Autodesk Inventor part; units mm, degrees
(part 2 of 2)
  spline S298 degree 2 poles (63.8368, 1.8656) (63.9127, 1.8656) (64.0147, 1.785) (64.0692, 1.6) (64.0977, 1.5668) knots 0 0 0 1 2 3 3 3
  spline S299 degree 2 poles (64.0977, 1.5668) (64.1593, 1.5004) (64.4676, 1.3676) (64.6503, 1.3676) knots 0 0 0 1 2 2 2
  spline S300 degree 2 poles (64.6503, 1.3676) (64.9372, 1.3676) (65.1222, 1.5004) knots 0 0 0 1 1 1
  spline S301 degree 2 poles (65.1222, 1.5004) (65.2384, 1.5834) (65.2384, 1.702) knots 0 0 0 1 1 1
  spline S302 degree 2 poles (65.2384, 1.702) (65.2384, 1.7826) (65.127, 1.9226) (64.9989, 1.9676) knots 0 0 0 1 2 2 2
  spline S303 degree 2 poles (64.9989, 1.9676) (64.9159, 1.9985) (64.6265, 2.053) knots 0 0 0 1 1 1
  spline S304 degree 2 poles (64.6265, 2.053) (64.2755, 2.1194) (63.9151, 2.302) (63.704, 2.6364) (63.704, 2.8309) knots 0 0 0 1 2 3 3 3
  spline S305 degree 2 poles (63.704, 2.8309) (63.704, 3.1392) (64.2186, 3.6017) (64.6313, 3.6017) knots 0 0 0 1 2 2 2
  spline S306 degree 2 poles (64.6313, 3.6017) (64.7973, 3.6017) (65.0795, 3.5281) (65.1957, 3.4523) knots 0 0 0 1 2 2 2
  spline S307 degree 2 poles (65.1957, 3.4523) (65.2787, 3.5353) (65.3641, 3.5353) knots 0 0 0 1 1 1
  spline S308 degree 2 poles (65.3641, 3.5353) (65.459, 3.5353) (65.5776, 3.4024) (65.5776, 3.2507) knots 0 0 0 1 2 2 2
  line L242 (65.5776, 3.2507) -> (65.5776, 2.9281)
  spline S309 degree 2 poles (65.5776, 2.9281) (65.5776, 2.774) (65.459, 2.6412) (65.3641, 2.6412) knots 0 0 0 1 2 2 2
  spline S310 degree 2 poles (65.3641, 2.6412) (65.2858, 2.6412) (65.2266, 2.6886) knots 0 0 0 1 1 1
  spline S311 degree 2 poles (65.2266, 2.6886) (65.1791, 2.7242) (65.1341, 2.9376) (65.0985, 2.985) knots 0 0 0 1 2 2 2
  spline S312 degree 2 poles (65.0985, 2.985) (65.0368, 3.0633) (64.7949, 3.1724) (64.636, 3.1724) knots 0 0 0 1 2 2 2
  spline S313 degree 2 poles (64.636, 3.1724) (64.4036, 3.1724) (64.1332, 2.9566) (64.1332, 2.8404) knots 0 0 0 1 2 2 2
  spline S314 degree 2 poles (64.1332, 2.8404) (64.1332, 2.7597) (64.2447, 2.6127) (64.3491, 2.57) knots 0 0 0 1 2 2 2
  spline S315 degree 2 poles (64.3491, 2.57) (64.4202, 2.5416) (65.0771, 2.4111) (65.4329, 2.257) (65.6677, 1.9249) (65.6677, 1.6973) knots 0 0 0 1 2 3 4 4 4
  spline S316 degree 2 poles (65.6677, 1.6973) (65.6677, 1.3795) (65.4447, 1.1897) knots 0 0 0 1 1 1
  spline S317 degree 2 poles (65.4447, 1.1897) (65.1459, 0.9383) (64.6858, 0.9383) knots 0 0 0 1 1 1
  spline S318 degree 2 poles (64.6858, 0.9383) (64.508, 0.9383) (64.1712, 1.0237) (64.0123, 1.1091) knots 0 0 0 1 2 2 2
  line L243 (67.4274, 3.1084) -> (67.4274, 1.4293)
  line L244 (67.4274, 1.4293) -> (67.8614, 1.4293)
  spline S319 degree 2 poles (67.8614, 1.4293) (68.0227, 1.4293) (68.1555, 1.3107) (68.1555, 1.2134) knots 0 0 0 1 2 2 2
  spline S320 degree 2 poles (68.1555, 1.2134) (68.1555, 1.1162) (68.0227, 1) (67.8614, 1) knots 0 0 0 1 2 2 2
  line L245 (67.8614, 1) -> (66.5642, 1)
  spline S321 degree 2 poles (66.5642, 1) (66.4029, 1) (66.2701, 1.1186) (66.2701, 1.2158) knots 0 0 0 1 2 2 2
  spline S322 degree 2 poles (66.2701, 1.2158) (66.2701, 1.3131) (66.4029, 1.4293) (66.5642, 1.4293) knots 0 0 0 1 2 2 2
  line L246 (66.5642, 1.4293) -> (66.9982, 1.4293)
  line L247 (66.9982, 1.4293) -> (66.9982, 3.1107)
  line L248 (66.9982, 3.1107) -> (66.5642, 3.1107)
  spline S323 degree 2 poles (66.5642, 3.1107) (66.4029, 3.1107) (66.2701, 3.2293) (66.2701, 3.3266) knots 0 0 0 1 2 2 2
  spline S324 degree 2 poles (66.2701, 3.3266) (66.2701, 3.4214) (66.4029, 3.54) (66.5642, 3.54) knots 0 0 0 1 2 2 2
  line L249 (66.5642, 3.54) -> (67.8614, 3.5376)
  spline S325 degree 2 poles (67.8614, 3.5376) (68.0227, 3.5376) (68.1555, 3.4214) (68.1555, 3.3242) knots 0 0 0 1 2 2 2
  spline S326 degree 2 poles (68.1555, 3.3242) (68.1555, 3.2269) (68.0227, 3.1084) (67.8614, 3.1084) knots 0 0 0 1 2 2 2
  line L250 (67.8614, 3.1084) -> (67.4274, 3.1084)
  line L251 (69.9935, 3.1107) -> (69.9935, 1.4293)
  line L252 (69.9935, 1.4293) -> (70.2828, 1.4293)
  spline S327 degree 2 poles (70.2828, 1.4293) (70.4441, 1.4293) (70.5769, 1.3107) (70.5769, 1.2134) knots 0 0 0 1 2 2 2
  spline S328 degree 2 poles (70.5769, 1.2134) (70.5769, 1.1162) (70.4441, 1) (70.2828, 1) knots 0 0 0 1 2 2 2
  line L253 (70.2828, 1) -> (69.2773, 1)
  spline S329 degree 2 poles (69.2773, 1) (69.116, 1) (68.9832, 1.1186) (68.9832, 1.2158) knots 0 0 0 1 2 2 2
  spline S330 degree 2 poles (68.9832, 1.2158) (68.9832, 1.3131) (69.116, 1.4293) (69.2773, 1.4293) knots 0 0 0 1 2 2 2
  line L254 (69.2773, 1.4293) -> (69.5642, 1.4293)
  line L255 (69.5642, 1.4293) -> (69.5642, 3.1107)
  line L256 (69.5642, 3.1107) -> (69.0994, 3.1107)
  line L257 (69.0994, 3.1107) -> (69.0994, 2.7052)
  spline S331 degree 2 poles (69.0994, 2.7052) (69.0994, 2.5439) (68.9808, 2.4111) (68.8836, 2.4111) knots 0 0 0 1 2 2 2
  spline S332 degree 2 poles (68.8836, 2.4111) (68.7864, 2.4111) (68.6701, 2.5439) (68.6701, 2.7052) knots 0 0 0 1 2 2 2
  line L258 (68.6701, 2.7052) -> (68.6701, 3.54)
  line L259 (68.6701, 3.54) -> (70.8947, 3.54)
  line L260 (70.8947, 3.54) -> (70.8947, 2.7052)
  spline S333 degree 2 poles (70.8947, 2.7052) (70.8947, 2.5439) (70.7761, 2.4111) (70.6789, 2.4111) knots 0 0 0 1 2 2 2
  spline S334 degree 2 poles (70.6789, 2.4111) (70.5817, 2.4111) (70.4655, 2.5439) (70.4655, 2.7052) knots 0 0 0 1 2 2 2
  line L261 (70.4655, 2.7052) -> (70.4655, 3.1107)
  line L262 (70.4655, 3.1107) -> (69.9935, 3.1107)
  line L263 (72.5762, 2.0649) -> (72.5762, 1.4293)
  line L264 (72.5762, 1.4293) -> (72.8655, 1.4293)
  spline S335 degree 2 poles (72.8655, 1.4293) (73.0268, 1.4293) (73.1596, 1.3107) (73.1596, 1.2134) knots 0 0 0 1 2 2 2
  spline S336 degree 2 poles (73.1596, 1.2134) (73.1596, 1.1162) (73.0268, 1) (72.8655, 1) knots 0 0 0 1 2 2 2
  line L265 (72.8655, 1) -> (71.8576, 1)
  spline S337 degree 2 poles (71.8576, 1) (71.6963, 1) (71.5635, 1.1186) (71.5635, 1.2158) knots 0 0 0 1 2 2 2
  spline S338 degree 2 poles (71.5635, 1.2158) (71.5635, 1.3131) (71.6963, 1.4293) (71.8576, 1.4293) knots 0 0 0 1 2 2 2
  line L266 (71.8576, 1.4293) -> (72.1469, 1.4293)
  line L267 (72.1469, 1.4293) -> (72.1469, 2.0649)
  line L268 (72.1469, 2.0649) -> (71.4354, 3.1131)
  spline S339 degree 2 poles (71.4354, 3.1131) (71.2742, 3.1131) (71.1414, 3.2317) (71.1414, 3.3289) knots 0 0 0 1 2 2 2
  spline S340 degree 2 poles (71.1414, 3.3289) (71.1414, 3.4238) (71.2742, 3.5424) (71.4354, 3.5424) knots 0 0 0 1 2 2 2
  line L269 (71.4354, 3.5424) -> (71.8386, 3.54)
  spline S341 degree 2 poles (71.8386, 3.54) (71.9952, 3.54) (72.128, 3.4238) (72.128, 3.3266) knots 0 0 0 1 2 2 2
  spline S342 degree 2 poles (72.128, 3.3266) (72.128, 3.1819) (71.9548, 3.1107) knots 0 0 0 1 1 1
  line L270 (71.9548, 3.1107) -> (72.3628, 2.5107)
  line L271 (72.3628, 2.5107) -> (72.7683, 3.1107)
  spline S343 degree 2 poles (72.7683, 3.1107) (72.607, 3.1107) (72.4742, 3.2293) (72.4742, 3.3266) knots 0 0 0 1 2 2 2
  spline S344 degree 2 poles (72.4742, 3.3266) (72.4742, 3.4214) (72.607, 3.54) (72.7683, 3.54) knots 0 0 0 1 2 2 2
  line L272 (72.7683, 3.54) -> (73.2853, 3.54)
  spline S345 degree 2 poles (73.2853, 3.54) (73.4442, 3.54) (73.577, 3.4238) (73.577, 3.3266) knots 0 0 0 1 2 2 2
  spline S346 degree 2 poles (73.577, 3.3266) (73.577, 3.2293) (73.4442, 3.1107) (73.2853, 3.1107) knots 0 0 0 1 2 2 2
  line L273 (73.2853, 3.1107) -> (72.5762, 2.0649)
  point P0 (10, -80)
  dimension "d0" = 20
  dimension "d1" = 5.4
  constraints: 1 horizontal
emboss "Top Label Text" sketch "Sketch4" operation cut depth 0.4 direction (0, 0, -1) contours L20 L21 S0 S1 L22 S2 S3 L23 L24 L25 S4 S5 L26 L27 S6 S7 L28 L29 L30 L31 S8 S9 S10 L32 S11 S12 S13 L33 | L34 S14 S15 L35 S16 S17 L36 S18 S19 L37 L38 S20 S21 S22 L39 L40 S23 S24 L41 S25 S26 | L42 L43 S27 S28 L44 L45 L46 L47 L48 L49 S29 S30 L50 L51 L52 L53 | L54 L55 S31 S32 L56 L57 L58 L59 L60 L61 S33 S34 L62 L63 L64 L65 | L66 L67 S35 S36 L68 S37 S38 L69 L70 L71 S39 S40 L72 S41 S42 L73 L74 S43 S44 L75 S45 S46 L76 | S47 S48 L77 S49 S50 S51 S52 S53 S54 S55 S56 S57 S58 S59 S60 L78 S61 S62 S63 S64 S65 S66 S67 S68 S69 S70 | L79 L80 S71 S72 L81 S73 S74 L82 L83 L84 S75 S76 L85 S77 S78 L86 L87 L88 S79 S80 L89 S81 S82 L90 S83 L91 S84 S85 L92 S86 S87 L93 | L94 L95 S88 S89 L96 S90 S91 L97 L98 L99 S92 S93 L100 S94 S95 L101 | L102 L103 S96 S97 L104 S98 S99 L105 L106 S100 S101 L107 L108 L109 L110 S102 S103 L111 S104 S105 L112 L113 L114 | L115 L116 S106 S107 L117 S108 S109 L118 L119 L120 L121 S110 S111 L122 L123 L124 S112 S113 L125 L126 | L127 L128 L129 S114 S115 L130 S116 S117 S118 L131 S119 S120 L132 S121 S122 L133 L134 L135 L136 L137 S123 S124 L138 S125 S126 L139 S127 S128 S129 L140 S130 S131 L141 L142 | L143 L144 S132 S133 L145 S134 S135 L146 L147 L148 S136 S137 L149 S138 S139 L150 | S140 S141 L151 S142 S143 S144 S145 S146 S147 L152 S148 S149 S150 S151 S152 S153 S154 S155 S156 S157 L153 S158 S159 | L154 L155 S160 S161 L156 S162 S163 L157 L158 L159 S164 S165 L160 S166 S167 L161 L162 L163 S168 S169 L164 S170 S171 L165 S172 L166 S173 S180 S179 S174 L167 S175 S176 L168 | S179 S180 S173 S174 | S174 S173 S180 L172 L173 S181 S182 L174 L175 L176 L177 S183 S184 L178 S185 S186 L179 L180 L181 L169 L170 S177 S178 L171 S179 | L182 L183 L184 S187 S188 L185 L186 S189 S190 L187 L188 L189 S191 S192 L190 L191 S193 S194 L192 L193 L194 L195 S195 S196 S197 L196 S198 S199 S200 S201 L197 | S202 S203 L198 S204 S205 S206 S207 S208 S209 S210 S211 S212 S213 S214 S215 L199 S216 S217 S218 S219 S220 S221 S222 S223 S224 S225 | S226 S227 L200 S228 S229 S230 S231 S232 S233 S234 S235 S236 S237 S238 S239 L201 S240 S241 S242 S243 S244 S245 S246 S247 S248 S249 | L202 S250 S251 S252 S253 L203 S254 S255 S256 S257 | L204 S258 S259 L205 S260 S261 L206 S262 S263 L207 S264 S265 | L212 L213 L214 S270 S271 L215 L216 S272 S273 L217 L218 L219 S274 S275 L220 L221 S276 S277 L222 L223 L224 L225 S278 S279 S280 L226 S281 S282 S283 S284 L227 | L228 L229 S285 S286 L230 S287 S288 L231 L232 S289 S290 L233 L234 L235 L236 S291 S292 L237 S293 S294 L238 L239 L240 | S295 S296 L241 S297 S298 S299 S300 S301 S302 S303 S304 S305 S306 S307 S308 L242 S309 S310 S311 S312 S313 S314 S315 S316 S317 S318 | L243 L244 S319 S320 L245 S321 S322 L246 L247 L248 S323 S324 L249 S325 S326 L250 | L251 L252 S327 S328 L253 S329 S330 L254 L255 L256 L257 S331 S332 L258 L259 L260 S333 S334 L261 L262 | L263 L264 S335 S336 L265 S337 S338 L266 L267 L268 S339 S340 L269 S341 S342 L270 L271 S343 S344 L272 S345 S346 L273
equation "\"d0\" = labelWidth"
equation "\"d1\" = labelThickness"
equation "\"d2\" = labelHeight"
equation "\"d4\" = tileWidth"
equation "\"d5\" = tileThickness"
equation "\"d6\" = tileWidth"
equation "\"d21\" = labelHeight"
equation "\"d22\" = labelThickness"
equation "\"d26\" = labelHeight"
equation "\"d10\" = tileSpacing"
equation "\"d35\" = tileSpacing"
equation "\"d38\" = tileSpacing"
equation "\"tileWidth\" = 15"
equation "\"tileThickness\" = 5"
equation "\"tileSpacing\" = tileWidth + tileThickness"
equation "\"labelWidth\" = tileWidth + labelHeight"
equation "\"labelHeight\" = 5"
equation "\"fuzzySkin_thicknessStart\" = 0.1"
equation "\"fuzzySkin_thicknessStep\" = 0.15"
equation "\"fuzzySkin_densityStart\" = 0.25"
equation "\"fuzzySkin_densityStep\" = 0.25"
equation "\"labelThickness\" = 5.4"
